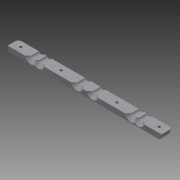
# Autodesk Inventor part: uhwyt przewodow przy zamknieciu
Saved by Autodesk Inventor 2014 (Build 180170000, 170)
## iProperties
Created: 2018-03-25
Part Number: uhwyt przewodow przy zamknieciu
Material: Generic
Document SubType Name: Modeling
Designer: HP820
Density: 1 g/cm^3
Appearance: Default
Author: HP820
Autodesk Inventor part; units mm, degrees
ref_plane "YZ Plane" through (0, 0, 0) normal (1, 0, 0) x (0, 1, 0)
ref_plane "XZ Plane" through (0, 0, 0) normal (0, 1, 0) x (-1, 0, 0)
ref_plane "XY Plane" through (0, 0, 0) normal (0, 0, 1) x (1, 0, 0)
sketch "Sketch1" plane through (0, 0, 0) normal (0, 1, 0) x (-1, 0, 0)
  line L0 (-100, 3.5) -> (100, 3.5)
  line L1 (100, 3.5) -> (100, -3.5)
  line L2 (100, -3.5) -> (-100, -3.5)
  line L3 (-100, -3.5) -> (-100, 3.5)
  line L4 (-100, 3.5) -> (100, -3.5) construction
  line L5 (100, 3.5) -> (-100, -3.5) construction
  point P0 (0, 0)
  dimension "d0" = 200
  dimension "d1" = 7
  constraints: 12 end point, 2 midpoint, 2 parallel, 1 horizontal, 1 perpendicular
  measures "d0" distance of L1.end L2.end
  measures "d1" distance of L0.end L1.end
extrude "Extrusion1" add sketch "Sketch1" along normal blind 14
sketch "Sketch2" plane through (0, 14, 0) normal (0, 1, 0) x (1, 0, 0)
  line L0 (100, 3.5) -> (-100, 3.5) projected
  line L1 (-100, 3.5) -> (-100, -3.5) projected
  circle A0 centre (-70, -5.25) radius 3.75
  circle A1 centre (-60, -5.25) radius 3.75
  circle A2 centre (-10, -5.25) radius 3.75
  circle A3 centre (10, -5.25) radius 3.75
  circle A4 centre (60, -5.25) radius 3.75
  circle A5 centre (70, -5.25) radius 3.75
  point P0 (0, 0)
  dimension "d4" = 7.5
  dimension "d5" = 7.5
  dimension "d6" = 30
  dimension "d7" = 40
  dimension "d8" = 8.75
  dimension "d9" = 8.75
  dimension "d10" = 7.5
  dimension "d11" = 7.5
  dimension "d12" = 7.5
  dimension "d13" = 7.5
  dimension "d14" = 90
  dimension "d15" = 110
  dimension "d16" = 160
  dimension "d17" = 170
  dimension "d20" = 8.75
  dimension "d21" = 8.75
  dimension "d22" = 8.75
  dimension "d23" = 8.75
  constraints: 6 centre point
  measures "d4" diameter of A0
  measures "d5" diameter of A1
  measures "d6" distance from line of L1 A0.centre
  measures "d7" distance from line of L1 A1.centre
  measures "d8" distance from line of L0 A0.centre
  measures "d9" distance from line of L0 A1.centre
  measures "d10" diameter of A2
  measures "d11" diameter of A3
  measures "d12" diameter of A4
  measures "d13" diameter of A5
  measures "d14" distance from line of L1 A2.centre
  measures "d15" distance from line of L1 A3.centre
  measures "d16" distance from line of L1 A4.centre
  measures "d17" distance from line of L1 A5.centre
  measures "d20" distance from line of L0 A2.centre
  measures "d21" distance from line of L0 A3.centre
  measures "d22" distance from line of L0 A4.centre
  measures "d23" distance from line of L0 A5.centre
extrude "Extrusion2" cut sketch "Sketch2" against normal up to surface (14 mm away)
sketch "Sketch4" plane through (100, 0, -3.5) normal (0, 0, -1) x (-1, 0, 0)
  line L0 (200, 0) -> (200, 14) projected
  line L1 (0, 0) -> (0, 14) projected
  circle A0 centre (10, 7) radius 1.7
  circle A1 centre (65, 7) radius 1.7
  circle A2 centre (137.5, 7) radius 1.7
  circle A3 centre (190, 7) radius 1.7
  point P0 (100, 0)
  dimension "d24" = 3.4
  dimension "d25" = 3.4
  dimension "d26" = 3.4
  dimension "d27" = 3.4
  dimension "d28" = 10
  dimension "d29" = 65
  dimension "d30" = 137.5
  dimension "d31" = 10
  constraints: 4 centre point
  measures "d24" diameter of A0
  measures "d25" diameter of A1
  measures "d26" diameter of A2
  measures "d27" diameter of A3
  measures "d28" distance from line of A0.centre L1
  measures "d29" distance from line of A1.centre L1
  measures "d30" distance from line of A2.centre L1
  measures "d31" distance from line of L0 A3.centre
extrude "Extrusion3" cut sketch "Sketch4" against normal blind 14
sketch "Sketch5" plane through (100, 0, -3.5) normal (0, 0, -1) x (-1, 0, 0)
  circle A0 centre (137.5, 7) radius 1.7 projected
  circle A1 centre (10, 7) radius 1.7 projected
  circle A2 centre (65, 7) radius 1.7 projected
  circle A3 centre (190, 7) radius 1.7 projected
  line L0 (13.695, 7) -> (11.8475, 3.8)
  line L1 (11.8475, 3.8) -> (8.1525, 3.8)
  line L2 (8.1525, 3.8) -> (6.305, 7)
  line L3 (6.305, 7) -> (8.1525, 10.2)
  line L4 (8.1525, 10.2) -> (11.8475, 10.2)
  line L5 (11.8475, 10.2) -> (13.695, 7)
  line L6 (66.8045, 10.2245) -> (68.6947, 7.0495)
  line L7 (68.6947, 7.0495) -> (66.8902, 3.825)
  line L8 (66.8902, 3.825) -> (63.1955, 3.7755)
  line L9 (63.1955, 3.7755) -> (61.3053, 6.9505)
  line L10 (61.3053, 6.9505) -> (63.1098, 10.175)
  line L11 (63.1098, 10.175) -> (66.8045, 10.2245)
  line L12 (139.357, 10.1945) -> (141.195, 6.989)
  line L13 (141.195, 6.989) -> (139.338, 3.7945)
  line L14 (139.338, 3.7945) -> (135.643, 3.8055)
  line L15 (135.643, 3.8055) -> (133.805, 7.011)
  line L16 (133.805, 7.011) -> (135.662, 10.2055)
  line L17 (135.662, 10.2055) -> (139.357, 10.1945)
  line L18 (191.8415, 10.2035) -> (193.695, 7.007)
  line L19 (193.695, 7.007) -> (191.8536, 3.8035)
  line L20 (191.8536, 3.8035) -> (188.1585, 3.7965)
  line L21 (188.1585, 3.7965) -> (186.305, 6.993)
  line L22 (186.305, 6.993) -> (188.1464, 10.1965)
  line L23 (188.1464, 10.1965) -> (191.8415, 10.2035)
  point P0 (100, 0)
  dimension "d34" = 6.4
  dimension "d35" = 6.4
  dimension "d36" = 6.4
  dimension "d37" = 6.4
  constraints: 48 end point, 4 coincident, 52 other
  measures "d34" distance between parallel lines of L20 L23
  measures "d35" distance between parallel lines of L14 L17
  measures "d36" distance between parallel lines of L8 L11
  measures "d37" distance between parallel lines of L1 L4
extrude "Extrusion4" cut sketch "Sketch5" against normal blind 2.4
chamfer "Chamfer1" distance 0.5 angle 45 24 edges at (-92.7743, 5.4052, -3.5) (-90.006, 3.8, -3.5) (-87.2317, 5.3948, -3.5) (-87.2257, 8.5948, -3.5) (-89.994, 10.2, -3.5) (-92.7683, 8.6052, -3.5) (-37.4905, 3.8, -3.5) (-40.2665, 5.3918, -3.5) (-40.276, 8.5918, -3.5) (-37.5095, 10.2, -3.5) (-34.7335, 8.6082, -3.5) (-34.724, 5.4082, -3.5) (35.0429, 10.1997, -3.5) (32.2504, 8.637, -3.5) (32.2075, 5.4373, -3.5) (34.9571, 3.8003, -3.5) (37.7496, 5.363, -3.5) (37.7925, 8.5627, -3.5) (90, 3.8, -3.5) (87.2287, 5.4, -3.5) (87.2287, 8.6, -3.5) (90, 10.2, -3.5) (92.7713, 8.6, -3.5) (92.7713, 5.4, -3.5)
chamfer "Chamfer2" distance 4 angle 45 6 edges at (-70, 0, 1.5) (-60, 0, 1.5) (-10, 0, 1.5) (10, 0, 1.5) (60, 0, 1.5) (70, 0, 1.5)
fillet "Fillet1" radius 4 5 edges at (-100, 7, -3.5) (-100, 14, 0) (0, 14, -3.5) (100, 14, 0) (100, 7, -3.5)
equation "\"d9\" = d8"
equation "\"d20\" = d8"
equation "\"d21\" = d20"
equation "\"d22\" = d21"
equation "\"d23\" = d21"
equation "\"d35\" = d34"
equation "\"d36\" = d35"
equation "\"d37\" = d36"
body "Solid1"
